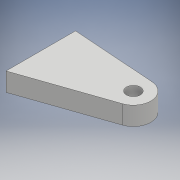
# Autodesk Inventor part: BaseHinge
Saved by Autodesk Inventor 2018.2 (Build 222227000, 227)
## iProperties
Created: 2018-03-04
Part Number: BaseHinge
Material: Generic
Document SubType Name: Modeling
Designer: Liam McNamee
Density: 1 g/cm^3
Appearance: Default
Author: Liam McNamee
Autodesk Inventor part; units mm, degrees
ref_plane "YZ Plane" through (0, 0, 0) normal (1, 0, 0) x (0, 1, 0)
ref_plane "XZ Plane" through (0, 0, 0) normal (0, 1, 0) x (-1, 0, 0)
ref_plane "XY Plane" through (0, 0, 0) normal (0, 0, 1) x (1, 0, 0)
sketch "Sketch1" plane through (0, 0, 0) normal (0, 0, 1) x (1, 0, 0)
  circle A0 centre (0, 0) radius 3
  arc A1 (2.4445, -7.0904) -> (0.5304, 7.4812) centre (0, 0) ccw
  line L0 (-35, 10) -> (-35, -20)
  line L1 (-35, 10) -> (0.5304, 7.4812)
  line L2 (-35, -20) -> (2.4445, -7.0904)
  dimension "d0" = 6
  dimension "d1" = 15
  dimension "d2" = 35
  dimension "d3" = 10
  dimension "d4" = 30
  constraints: 6 end point, 2 centre point, 2 coincident, 2 point on circle, 2 tangent, 1 vertical
  measures "d0" diameter of A0
  measures "d1" diameter of A1
  measures "d2" distance from line of point (0, 0) L0
  measures "d3" vertical distance of point (0, 0) L0.start
  measures "d4" distance of L0.start L0.end
extrude "Extrusion1" add sketch "Sketch1" against normal blind 8
body "Solid1"
